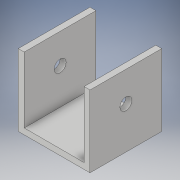
# Autodesk Inventor part: CLB_062_ScissorLiftUBracket
Saved by Autodesk Inventor 2018.3 (Build 223284000, 284)
## iProperties
Created: 2020-01-25
Part Number: CLB_062_ScissorLiftUBracket
Material: Generic
Document SubType Name: Modeling
Designer: Cooper
Density: 1 g/cm^3
Appearance: Default
Author: Cooper
Autodesk Inventor part; units mm, degrees
ref_plane "YZ Plane" through (0, 0, 0) normal (1, 0, 0) x (0, 1, 0)
ref_plane "XZ Plane" through (0, 0, 0) normal (0, 1, 0) x (-1, 0, 0)
ref_plane "XY Plane" through (0, 0, 0) normal (0, 0, 1) x (1, 0, 0)
sketch "Sketch1" plane through (0, 0, 0) normal (0, 0, 1) x (1, 0, 0)
  line L0 (0, 0) -> (0, 38.1)
  line L1 (0, 38.1) -> (3.175, 38.1)
  line L2 (3.175, 38.1) -> (3.175, 3.175)
  line L3 (3.175, 3.175) -> (34.925, 3.175)
  line L4 (34.925, 3.175) -> (34.925, 38.1)
  line L5 (34.925, 38.1) -> (38.1, 38.1)
  line L6 (38.1, 38.1) -> (38.1, 0)
  line L7 (38.1, 0) -> (0, 0)
  dimension "d0" = 38.1
  dimension "d2" = 3.175
  dimension "d3" = 3.175
  dimension "d4" = 38.1
  dimension "d5" = 3.175
  constraints: 16 end point, 6 perpendicular, 2 point on line, 1 vertical
  measures "d0" distance of L6.end L0.start
  measures "d2" distance between parallel lines of L2 L0
  measures "d3" distance between parallel lines of L6 L4
  measures "d4" distance of L0.start L0.end
  measures "d5" distance between parallel lines of L7 L3
extrude "Extrusion1" add sketch "Sketch1" along normal blind 38.1
sketch "Sketch2" plane through (38.1, 0, 0) normal (1, 0, 0) x (0, 0, -1)
  line L0 (0, 38.1) -> (0, 0) projected
  line L1 (0, 38.1) -> (-38.1, 38.1) projected
  line L2 (-38.1, 0) -> (-38.1, 38.1) projected
  line L3 (0, 0) -> (-38.1, 0) projected
  line L4 (0, 3.175) -> (-38.1, 3.175) projected
  point P0 (0, 0)
  point P1 (-19.05, 22.225)
  dimension "d8" = 19.05
  dimension "d9" = 19.05
  dimension "d19" = 19.05
  measures "d8" distance from line of point (-19.05, 22.225) L2
  measures "d9" distance from line of L0 point (-19.05, 22.225)
  measures "d19" distance from line of L4 point (-19.05, 22.225)
hole "Hole1" at (38.1, 22.225, 19.05) direction (-1, 0, 0) diameter 6.35 end through all
equation "\"d3\" = d2"
equation "\"d5\" = d2"
equation "\"d8\" = d9"
body "Solid1"
